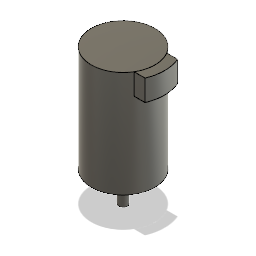
Motor (Autodesk Fusion 360 design; units mm, degrees)
Autodesk Fusion 360 part; units mm, degrees
sketch "Sketch1" plane through (0, 0, 0) normal (0, 1, 0) x (1, 0, 0)
  circle A0 centre (0, 0) radius 18
  dimension "d1" = 36
  constraint coincident A0.centre origin
  measures "d1" diameter of A0
extrude "Extrude1" add sketch "Sketch1" along normal blind 60 makes body 1
sketch "Sketch2" plane through (0, 0, 0) normal (0, -1, 0) x (1, 0, 0)
  circle A0 centre (0, 0) radius 18
  circle A1 centre (0, 0) radius 2.5
  dimension "d4" = 5
  constraint coincident A0.centre A1.centre
  measures "d4" diameter of A1
extrude "Extrude2" add sketch "Sketch2" along normal blind 17 contours A1 bodies 1
sketch "Sketch3" plane through (0, 60, 0) normal (0, 1, 0) x (-1, 0, 0)
  circle A0 centre (0, 0) radius 18
  arc A1 (-21.603, 9.25) -> (-21.603, -9.25) centre (0, 0) ccw
  line L0 (-21.603, -9.25) -> (-15.4407, -9.2513)
  line L1 (-21.603, 9.25) -> (-15.4408, 9.2511)
  dimension "d7" = 23.5
  dimension "d8" = 18.5
  dimension "d9" = 6.1623
  dimension "d10" = 6.1622
  constraint coincident A0.centre A1.centre
  constraint vertical A1.start A1.end
  constraint coincident A0 L0.end
  constraint coincident A0 L1.end
  measures "d7" radius of A1
  measures "d8" distance of A1.start A1.end
  measures "d9" horizontal distance of A1.end L0.end
  measures "d10" horizontal distance of A1.start L1.end
extrude "Extrude3" add sketch "Sketch3" against normal blind 12 separate body contours A0 A1 L0 L1 makes body 2
